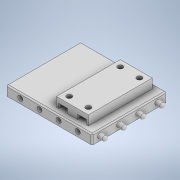
# Autodesk Inventor part: test attatchment
Saved by Autodesk Inventor 2022 (Build 260153000, 153)
## iProperties
Created: 2021-11-12
Part Number: test attatchment
Material: Generic
Document SubType Name: Modeling
Designer: a-dubs
Density: 1 g/cm^3
Appearance: Default
Author: a-dubs
Autodesk Inventor part; units mm, degrees
ref_plane "YZ Plane" through (0, 0, 0) normal (1, 0, 0) x (0, 1, 0)
ref_plane "XZ Plane" through (0, 0, 0) normal (0, 1, 0) x (-1, 0, 0)
ref_plane "XY Plane" through (0, 0, 0) normal (0, 0, 1) x (1, 0, 0)
derived "backplate reinforcementipt.ipt"
sketch "Sketch2" plane through (-84.25, 0, 90.5981) normal (-1, 0, 0) x (0, 0, 1)
  line L0 (68.7, 0) -> (68.7, 6)
  line L1 (0, 0) -> (68.7, 0)
  line L2 (68.7, 0) -> (68.7, 6)
  line L3 (68.7, 6) -> (0, 6)
  line L4 (0, 6) -> (0, 0)
  line L5 (0, 0) -> (0, 6)
  line L6 (0, 3) -> (2.35, 3)
  line L7 (34.3, 0) -> (34.3, 6)
  line L8 (34.3, 6) -> (34.3, 0)
  line L9 (68.6, 3) -> (66.25, 3)
  line L10 (2.35, 3) -> (3.95, 3)
  circle A0 centre (3.95, 3) radius 1.6
  circle A1 centre (15.95, 3) radius 1.6
  circle A2 centre (27.95, 3) radius 1.6
  circle A3 centre (39.95, 3) radius 1.6
  circle A4 centre (51.95, 3) radius 1.6
  circle A5 centre (63.95, 3) radius 1.6
  circle A6 centre (63.95, 3) radius 1.45
  circle A7 centre (51.95, 3) radius 1.45
  circle A8 centre (39.95, 3) radius 1.45
  circle A9 centre (27.95, 3) radius 1.45
  circle A10 centre (15.95, 3) radius 1.5
  circle A11 centre (3.95, 3) radius 1.5
  line L11 (27.95, 3) -> (21.95, 3)
  line L12 (21.95, 3) -> (21.95, 6)
  line L13 (21.95, 0) -> (21.95, 3)
  point P0 (-90.5981, 0)
  dimension "d47" = 12
  dimension "d6" = 2.9
  dimension "d7" = 2.9
  dimension "d8" = 2.9
  dimension "d9" = 2.9
  dimension "d10" = 3
  dimension "d11" = 3
  dimension "d42" = 6
  measures "d6" diameter of A6
  measures "d7" diameter of A7
  measures "d8" diameter of A8
  measures "d9" diameter of A9
  measures "d10" diameter of A10
  measures "d11" diameter of A11
  measures "d42" distance of L11.start L11.end
extrude "Extrusion1" add sketch "Sketch2" along normal blind 54 contours L1 L7 L3 L0 | L1 L13 L12 L3 L7 | A2 | A3 | A4 | A5 | A6 | A7 | A8 | A9
extrude "Extrusion2" add sketch "Sketch2" against normal blind 4.5 contours A6 | A7 | A8 | A9
fillet "Fillet1" radius 1.45 4 edges at (-79.75, 3, 153.0981) (-79.75, 3, 141.0981) (-79.75, 3, 129.0981) (-79.75, 3, 117.0981)
chamfer "Chamfer1" distance 0.75 angle 45 4 edges at (-111.25, 6, 159.2981) (-84.25, 6, 135.9231) (-138.25, 6, 135.9231) (-111.25, 6, 112.5481)
fillet "Fillet2" radius 1 4 edges at (-138.25, 2.625, 159.2981) (-84.25, 2.625, 159.2981) (-138.25, 2.625, 112.5481) (-84.25, 2.625, 112.5481)
sketch "Sketch3" plane through (-85.25, 5.25, 159.2981) normal (0, 0, -1) x (-1, 0, 0)
  line L0 (0, 0) -> (0, -5.25) projected
  line L1 (0, -2.625) -> (8, -2.625)
  circle A0 centre (8, -2.625) radius 1.6
  circle A1 centre (20, -2.625) radius 1.6
  circle A2 centre (32, -2.625) radius 1.6
  circle A3 centre (44, -2.625) radius 1.6
  line L2 (0, -5.25) -> (52, -5.25) projected
  line L3 (0, -5.25) -> (0, 0.75)
  line L4 (0, 0.75) -> (0, -2.25)
  line L5 (0, -5.25) -> (0, 0) projected
  line L6 (0, -2.25) -> (8, -2.25)
  circle A4 centre (8, -2.25) radius 1.6
  circle A5 centre (20, -2.25) radius 1.6
  circle A6 centre (32, -2.25) radius 1.6
  circle A7 centre (44, -2.25) radius 1.6
  point P0 (-85.25, -5.25)
  point P1 (6.4, -2.25)
  point P2 (6.4446, -2.25)
  point P3 (6.411, -2.4375)
  point P4 (6.4446, -2.625)
  point P5 (6.4, -2.625)
  dimension "d16" = 8
  dimension "d17" = 3.2
  dimension "d20" = 12
  dimension "d31" = 6
  dimension "d32" = 3
  dimension "d33" = 8
  dimension "d34" = 3.2
  dimension "d37" = 12
  constraints: 8 centre point, 8 end point, 4 horizontal, 2 coincident, 1 midpoint, 1 point on line, 1 vertical, 12 other
  measures "d16" distance of L1.start L1.end
  measures "d17" diameter of A0
  measures "d20" distance of A0.centre A1.centre
  measures "d31" distance of L0.end L3.end
  measures "d32" distance of L3.end L4.end
  measures "d33" distance of L4.end L6.end
  measures "d34" diameter of A4
  measures "d37" distance of A4.centre A5.centre
extrude "Extrusion3" cut sketch "Sketch3" against normal blind 5 from surface at 46.75 contours A4 A0 L6 | L6 A0 A4 | A0 A4 | A5 A1 | A1 A5 | A6 A2 | A2 A6 | A7 A3 | A3 A7 picked at (19.8721, -2.8928) picked at (20.2203, -0.9236) picked at (31.8721, -2.8928) picked at (32.2203, -0.9236) picked at (43.8721, -1.9822) picked at (44.2203, -0.9236)
extrude "Extrusion4" cut sketch "Sketch3" along normal blind 5 from surface at 0 contours A4 A0 L6 | L6 A0 A4 | A0 A4 | A5 A1 | A1 A5 | A6 A2 | A2 A6 | A7 A3 | A3 A7 picked at (19.8721, -2.8928) picked at (20.2203, -0.9236) picked at (31.8721, -2.8928) picked at (32.2203, -0.9236) picked at (43.8721, -1.9822) picked at (44.2203, -0.9236)
extrude "Extrusion5" cut sketch "Sketch2" against normal blind 4.5 from surface at 54 contours A0 | A1 | A2 | A3 | A4 | A5 | A6 | A7 | A8 | A9 | A10 | A11
sketch "Sketch4" plane through (-137.5, 6, 158.5481) normal (0, 1, 0) x (1, 0, 0)
  line L0 (0, 0) -> (0, 45.25) projected
  line L1 (0, 45.25) -> (0, 0)
  line L2 (0, 0) -> (52.5672, 0)
  line L3 (52.5, 45.25) -> (52.5, 0) projected
  line L4 (52.5, 0) -> (52.5, 45.25)
  line L5 (52.5, 22.625) -> (47.5, 22.625)
  line L6 (47.5, 22.625) -> (47.5, 42.625)
  line L7 (47.5, 22.625) -> (47.5, 2.625)
  line L8 (47.5, 42.625) -> (27.5, 42.625)
  line L9 (27.5, 42.625) -> (27.5, 2.625)
  line L10 (27.5, 2.625) -> (47.5, 2.625)
  line L11 (47.5, 22.625) -> (47.5, 10.625)
  line L12 (47.5, 22.625) -> (27.5, 22.625)
  line L13 (47.5, 22.625) -> (47.5, 34.625)
  line L14 (47.5, 10.625) -> (27.5, 10.625)
  line L15 (47.5, 34.625) -> (27.5, 34.625)
  line L16 (47.5, 10.625) -> (47.5, 2.625)
  line L17 (47.5, 2.625) -> (43.5, 2.625)
  line L18 (43.5, 2.625) -> (43.5, 6.625)
  line L19 (27.5, 2.625) -> (31.5, 2.625)
  line L20 (31.5, 2.625) -> (31.5, 6.625)
  circle A0 centre (31.5, 6.625) radius 1.6
  circle A1 centre (43.5, 6.625) radius 1.6
  circle A2 centre (31.5, 38.625) radius 1.6
  circle A3 centre (43.5, 38.625) radius 1.6
  line L21 (27.5, 2.625) -> (25.5, 2.625)
  line L22 (25.5, 2.625) -> (25.5, 0.625)
  line L23 (47.5, 42.625) -> (47.5, 44.625)
  line L24 (47.5, 44.625) -> (49.5, 44.625)
  line L25 (25.5, 0.625) -> (49.5, 0.625)
  line L26 (49.5, 0.625) -> (49.5, 44.625)
  line L27 (49.5, 44.625) -> (25.5, 44.625)
  line L28 (25.5, 44.625) -> (25.5, 0.625)
  line L29 (43.5, 6.625) -> (40.7, 6.625)
  line L30 (40.7, 6.625) -> (40.7, 3.825)
  line L31 (40.7, 3.825) -> (43.5, 3.825)
  line L32 (43.5, 3.825) -> (43.5, 6.625)
  line L33 (40.7, 3.825) -> (46.3, 3.825)
  line L34 (46.3, 3.825) -> (46.3, 9.425)
  line L35 (46.3, 9.425) -> (40.7, 9.425)
  line L36 (40.7, 9.425) -> (40.7, 3.825)
  line L37 (40.7, 41.425) -> (43.5, 41.425)
  line L38 (40.7, 41.425) -> (46.3, 41.425)
  line L39 (46.3, 41.425) -> (46.3, 35.825)
  line L40 (46.3, 35.825) -> (40.7, 35.825)
  line L41 (40.7, 35.825) -> (40.7, 41.425)
  line L42 (27.5, 2.625) -> (47.5, 2.625)
  line L43 (37.5, 2.625) -> (37.5, 42.625)
  line L44 (34.3, 3.825) -> (28.7, 3.825)
  line L45 (28.7, 3.825) -> (28.7, 9.425)
  line L46 (28.7, 9.425) -> (34.3, 9.425)
  line L47 (34.3, 9.425) -> (34.3, 3.825)
  line L48 (28.7, 35.825) -> (34.3, 35.825)
  line L49 (34.3, 35.825) -> (34.3, 41.425)
  line L50 (34.3, 41.425) -> (28.7, 41.425)
  line L51 (28.7, 41.425) -> (28.7, 35.825)
  line L52 (28.7, 3.825) -> (28.7, 2.625)
  line L53 (34.3, 3.825) -> (34.3, 2.625)
  line L54 (46.3, 3.825) -> (46.3, 2.625)
  line L55 (40.7, 3.825) -> (40.7, 2.625)
  line L56 (46.3, 41.425) -> (46.3, 42.625)
  line L57 (40.7, 41.425) -> (40.7, 42.625)
  line L58 (28.7, 41.425) -> (28.7, 42.625)
  line L59 (34.3, 41.425) -> (34.3, 42.625)
  point P0 (137.5, 158.5481)
  point P1 (26.2836, 22.625)
  point P2 (34.3, 2.625)
  point P3 (40.7, 2.625)
  point P4 (40.7, 6.625)
  point P5 (46.3, 2.625)
  point P6 (28.7, 2.625)
  dimension "d43" = 5
  dimension "d44" = 20
  dimension "d45" = 20
  dimension "d46" = 12
  dimension "d47" = 12
  dimension "d48" = 4
  dimension "d49" = 4
  dimension "d50" = 3.2
  dimension "d56" = 2
  dimension "d57" = 2
  dimension "d58" = 2
  dimension "d59" = 2
  dimension "d60" = 2.8
  dimension "d61" = 2.8
  dimension "d62" = 5.6
  dimension "d63" = 5.6
  constraints: 116 end point, 17 perpendicular, 17 point on line, 15 symmetric about line, 6 parallel, 5 collinear, 5 horizontal, 4 centre point, 4 midpoint, 4 vertical, 2 coincident, 1 equal radius, 2 other
  measures "d43" distance of L5.start L5.end
  measures "d44" distance of L5.end L6.end
  measures "d45" distance of L6.end L8.end
  measures "d46" distance of L5.end L11.end
  measures "d47" distance of L5.end L13.end
  measures "d48" distance of L7.end L17.end
  measures "d49" distance of L9.end L19.end
  measures "d50" diameter of A0
  measures "d56" distance of L9.end L21.end
  measures "d57" distance of L21.end L22.end
  measures "d58" distance of L6.end L23.end
  measures "d59" distance of L23.end L24.end
  measures "d60" distance of L31.end L30.end
  measures "d61" distance of L30.end L29.end
  measures "d62" distance of L35.end L34.end
  measures "d63" distance of L34.end L33.end
extrude "Extrusion6" add sketch "Sketch4" along normal blind 3 contours L12 L43 L15 L6 | L7 L14 L43 L12 | L15 L43 L8 L57 L41 L40 L39 L56 L6 | L7 L10 L54 L34 L35 L36 L30 L55 L43 L14 | L43 L14 L9 L12 | L12 L9 L15 L43 | L15 L9 L8 L58 L51 L48 L49 L59 L43 | L43 L10 L53 L47 L46 L45 L52 L9 L14
extrude "Extrusion7" add sketch "Sketch4" along normal blind 3 from surface at 3 contours L12 L43 L15 L6 | L7 L14 L43 L12 | L15 L43 L8 L57 L41 L40 L39 L56 L6 | L7 L10 L54 L34 L35 L36 L30 L55 L43 L14 | L43 L14 L9 L12 | L12 L9 L15 L43 | L15 L9 L8 L58 L51 L48 L49 L59 L43 | L43 L10 L53 L47 L46 L45 L52 L9 L14 | L56 L38 L37 L57 L8 | L10 L18 L33 L54 | L39 L40 L41 L37 L38 | L59 L50 L58 L8 | L10 L55 L31 L18 | L33 L18 A1 L29 L36 L35 L34 | L10 L20 L44 L53 | L52 L44 L20 L10 | L49 L48 L51 L50 | L31 L30 L29 A1 L18 | L44 L45 L46 L47
body "Solid1"
